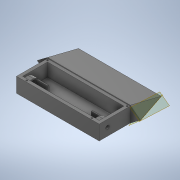
# Autodesk Inventor part: BodyWedgeV3
Saved by Autodesk Inventor 2020 (Build 240168000, 168)
## iProperties
Created: 2023-11-26
Part Number: BodyWedgeV3
Material: Thermoplastic Resin
Document SubType Name: Modeling
Designer: smz3rm
Density: 1.28 g/cm^3
Appearance: Smooth - Black
Mass: 333.31 g
Surface Area: 631.422 cm^2
Volume: 260.399 cm^3
Author: smz3rm
Autodesk Inventor part; units mm, degrees
ref_plane "YZ Plane" through (0, 0, 0) normal (1, 0, 0) x (0, 1, 0)
ref_plane "XZ Plane" through (0, 0, 0) normal (0, 1, 0) x (-1, 0, 0)
sketch "Sketch1" plane through (0, 0, 0) normal (0, 1, 0) x (-1, 0, 0)
  line L0 (80, 30) -> (-80, 30)
  line L1 (-80, 30) -> (-80, -30)
  line L2 (-80, -30) -> (80, -30)
  line L3 (80, -30) -> (80, 30)
  line L4 (80, 30) -> (-80, -30) construction
  line L5 (-80, 30) -> (80, -30) construction
  line L6 (0, -42) -> (0, 42) projected
  point P0 (0, 0)
  point P1 (-100, -30)
  point P2 (-80, -27)
  dimension "d0" = 160
  dimension "d1" = 60
  dimension "d32" = 20
  constraints: 12 end point, 2 midpoint, 2 parallel, 2 point on line, 1 horizontal, 1 perpendicular
  measures "d0" distance of L2.end L1.end
  measures "d1" distance of L1.end L0.end
  measures "d32" distance of L1.end point (-100, -30)
extrude "Extrusion1" add sketch "Sketch1" along normal blind 3
sketch "Sketch2" plane through (0, 3, 0) normal (0, 1, 0) x (1, 0, 0)
  line L0 (-80, 30) -> (-80, -30) projected
  line L1 (-80, -30) -> (80, -30) projected
  line L2 (80, -30) -> (80, 30) projected
  line L3 (74, -24) -> (-74, -24)
  line L4 (-74, -24) -> (-74, 24)
  line L5 (-74, 24) -> (74, 24)
  line L6 (74, 24) -> (74, -24)
  line L7 (74, -24) -> (-74, 24) construction
  line L8 (-74, -24) -> (74, 24) construction
  line L9 (80, 30) -> (-80, 30) projected
  point P0 (0, 0)
  dimension "d36" = 148
  dimension "d37" = 48
  constraints: 12 end point, 2 midpoint, 2 parallel, 1 horizontal, 1 perpendicular
  measures "d36" distance of L4.end L5.end
  measures "d37" distance between parallel lines of L5 L3
extrude "Extrusion2" add sketch "Sketch2" along normal blind 24
sketch "Sketch7" plane through (-74, 3, 24) normal (1, 0, 0) x (0, 0, -1)
  circle A0 centre (10, 12) radius 8
  line L0 (54, -3) -> (-6, -3) projected
  circle A1 centre (10, 12) radius 10
  line L1 (0, 12) -> (0, 0)
  line L2 (0, 12) -> (20, 12)
  line L3 (20, 12) -> (20, 0)
  line L4 (-6, -3) -> (-6, 24) projected
  line L5 (0, 0) -> (20, 0)
  line L6 (10, 22) -> (0, 22)
  line L7 (0, 0) -> (0, 24) projected
  line L8 (0, 12) -> (0, 22)
  point P0 (24, -3)
  point P1 (54, -3)
  dimension "MotorDiameter" = 16
  dimension "d18" = 15
  dimension "d20" = 2
  dimension "d40" = 20
  dimension "d62" = 10
  constraints: 12 end point, 3 horizontal, 3 point on circle, 2 centre point, 2 vertical, 1 perpendicular, 1 point on line
  measures "MotorDiameter" diameter of A0
  measures "d18" distance from line of L0 A0.centre
  measures "d20" radial gap between concentric circles of A0 A1
  measures "d40" distance between parallel lines of L3 L1
  measures "d62" distance of L6.start L6.end
extrude "Extrusion5" add sketch "Sketch7" along normal blind 11.25 contours L2 A1 A0 | A0 L2 A1 | L3 L5 L1 A1 | L7 L6 A1
sketch "Sketch8" plane through (-62.75, 3, 24) normal (1, 0, 0) x (0, 0, -1)
  arc A0 (20, 12) -> (10, 22) centre (10, 12) ccw projected
  circle A1 centre (10, 12) radius 8 projected
  line L0 (0, 0) -> (0, 22) projected
  line L1 (20, 0) -> (0, 0) projected
  line L2 (20, 0) -> (20, 12) projected
  circle A2 centre (10, 12) radius 7.75
  line L3 (10, 22) -> (0, 22) projected
  line L4 (0, 0) -> (0, 22) projected
  line L5 (4, 7.0946) -> (4, 17.2915)
  line L6 (10, 22) -> (0, 22) projected
  line L7 (16, 7.0946) -> (16, 17.2915)
  line L8 (16, 17.2915) -> (18.4853, 17.2915)
  arc A3 (20, 12) -> (10, 22) centre (10, 12) ccw projected
  line L9 (4, 17.2915) -> (0, 17.2915)
  point P0 (24, -3)
  point P1 (4, 27)
  point P2 (4, 16.9054)
  point P3 (16, 16.9054)
  dimension "d55" = 15.5
  dimension "d63" = 12
  dimension "d64" = 6
  constraints: 8 end point, 6 point on circle, 2 coincident, 2 perpendicular, 2 point on line, 1 centre point, 1 horizontal, 1 vertical
  measures "d55" diameter of A2
  measures "d63" distance between parallel lines of L7 L5
  measures "d64" distance from line of L5 point (10, 12)
extrude "Extrusion6" add sketch "Sketch8" along normal blind 20 contours L2 L1 L0 L9 A1 L8 A0 | A1 L5 A2 L7 | A2 L7 | L5 A2 picked at (9.114, 4.2488)
sketch "Sketch9" plane through (-74, 20, 20) normal (1, 0, 0) x (0, 0, -1)
  circle A0 centre (6, -5) radius 3.5
  line L0 (50, -20) -> (-10, -20) projected
  line L1 (-10, -20) -> (-10, 7) projected
  point P0 (20, -20)
  point P1 (44, -20)
  dimension "d27" = 7
  dimension "d28" = 15
  dimension "d41" = 16
  constraints: 1 centre point
  measures "d27" diameter of A0
  measures "d28" distance from line of L0 A0.centre
  measures "d41" distance from line of L1 A0.centre
extrude "Extrusion7" cut sketch "Sketch9" against normal up to surface (6 mm away)
mirror "Mirror2" about plane through (0, 0, 0) normal (1, 0, 0) of "Extrusion7", "Extrusion6", "Extrusion5"
sketch "Sketch15" plane through (80, 0, 30) normal (1, 0, 0) x (0, 0, -1)
  line L0 (60, 27) -> (0, 27) projected
  circle A0 centre (16, 15) radius 3.5 projected
  line L1 (0, 0) -> (60, 0) projected
  line L2 (60, 0) -> (60, 27) projected
  line L3 (0, 27) -> (60, 27) projected
  line L4 (0, 0) -> (0, 27) projected
  line L5 (60, 0) -> (60, 27) projected
  line L6 (120.0188, 15.0047) -> (60, 0)
  line L7 (60, 0) -> (60, 27) projected
  line L8 (60, 0) -> (60, 30)
  line L9 (60, 15) -> (120, 15)
  line L10 (60, 30) -> (120, 15)
  point P0 (30, 0)
  dimension "d104" = 30
  dimension "d105" = 15
  dimension "d106" = 60
  constraints: 8 end point, 1 horizontal, 1 midpoint, 1 point on line, 1 vertical
  measures "d104" distance of L1.end L8.end
  measures "d105" distance of L8.end L9.start
  measures "d106" distance of L9.start L9.end
extrude "Extrusion18" add sketch "Sketch15" against normal up to surface (160 mm away) contours L8 L10 L9 L2 | L9 L6 L2
ref_plane "Work Plane9" through (79, -4, -30) normal (0, 0, -1) x (-1, 0, 0)
sketch "Sketch23" plane through (79, -4, -30) normal (0, 0, -1) x (-1, 0, 0)
  line L0 (-1, 34) -> (-21, 19)
  line L1 (-21, 19) -> (-1, 19)
  line L2 (-21, 19) -> (-1, 4)
  line L3 (-1, 31) -> (159, 31) projected
  line L4 (-1, 34) -> (-1, 31) projected
  line L5 (-1, 34) -> (159, 34) projected
  line L6 (159, 34) -> (159, 31) projected
  line L7 (159, 4) -> (-1, 4) projected
  line L8 (-1, 4) -> (-1, 31) projected
  line L9 (159, 31) -> (-1, 31) projected
  line L10 (159, 4) -> (159, 31) projected
  point P0 (79, 4)
  dimension "d97" = 20
  dimension "d108" = 15
  constraints: 6 end point, 1 horizontal, 1 point on line
  measures "d97" distance of L0.end L1.end
  measures "d108" distance of L0.start L1.end
extrude "Extrusion19" add sketch "Sketch23" along normal blind 60 contours L4 L8 L1 L0 | L1 L8 L2
ref_plane "Work Plane4" through (100, 15, -30) normal (-0.5883, -0.7845, 0.1961) x (-0.8, 0.6, 0)
sketch "Sketch24" plane through (100, 15, -30) normal (-0.5883, -0.7845, 0.1961) x (-0.8, 0.6, 0)
  line L0 (-89.1969, -73.3175) -> (145.8797, -73.3175)
  line L1 (145.8797, -73.3175) -> (145.8797, 67.3582)
  line L2 (145.8797, 67.3582) -> (-89.1969, 67.3582)
  line L3 (-89.1969, 67.3582) -> (-89.1969, -73.3175)
  point P0 (71, -15.2971)
  constraints: 8 end point, 2 parallel, 1 horizontal, 1 perpendicular
extrude "Extrusion20" cut sketch "Sketch24" against normal blind 60
ref_plane "Work Plane5" through (80, 15, -90) normal (0.5883, -0.7845, -0.1961) x (0.3162, 0, 0.9487)
sketch "Sketch25" plane through (80, 15, -90) normal (0.5883, -0.7845, -0.1961) x (0.3162, 0, 0.9487)
  line L0 (-115.6054, 99.2741) -> (196.6383, 99.2741)
  line L1 (196.6383, 99.2741) -> (196.6383, -110.1424)
  line L2 (196.6383, -110.1424) -> (-115.6054, -110.1424)
  line L3 (-115.6054, -110.1424) -> (-115.6054, 99.2741)
  point P0 (60.0833, 91.1655)
  constraints: 8 end point, 2 parallel, 1 horizontal, 1 perpendicular
extrude "Extrusion21" cut sketch "Sketch25" along normal blind 60
mirror "Mirror10" about plane through (0, 0, 0) normal (1, 0, 0) of "Extrusion19", "Extrusion20", "Extrusion21"
sketch "Sketch26" plane through (0, 27, 0) normal (0, 1, 0) x (1, 0, 0)
  line L0 (-80, 30) -> (-80, -30) projected
  line L1 (-80, -30) -> (80, -30) projected
  line L2 (80, -30) -> (80, 30) projected
  line L3 (80, 30) -> (-80, 30) projected
  line L4 (-74, 24) -> (74, 24) projected
  line L5 (74, 24) -> (74, -24) projected
  line L6 (74, -24) -> (-74, -24) projected
  line L7 (-74, -24) -> (-74, 24) projected
  point P0 (0, 0)
extrude "Extrusion22" add sketch "Sketch26" along normal blind 1.4125
sketch "Sketch27" plane through (0, 28.4125, 0) normal (0, 1, 0) x (1, 0, 0)
  line L0 (-80, 30) -> (-80, -30) projected
  line L1 (-80, -30) -> (80, -30) projected
  line L2 (80, -30) -> (80, 30) projected
  line L3 (-80, 30) -> (80, 30) projected
  line L4 (-74, -24) -> (-74, 24) projected
  line L5 (-74, 24) -> (74, 24) projected
  line L6 (74, 24) -> (74, -24) projected
  line L7 (74, -24) -> (-74, -24) projected
  line L8 (80, -30) -> (80, 30) projected
  line L9 (80, -27) -> (-80, -27)
  line L10 (-80, 30) -> (-80, -30) projected
  line L11 (80, 27) -> (-80, 27)
  line L12 (-80, -30) -> (80, -30) projected
  line L13 (77, -30) -> (77, 30)
  circle A0 centre (63, -27) radius 1.45
  circle A1 centre (77, 27) radius 1.45
  line L14 (0, 114) -> (0, -54) projected
  circle A2 centre (-63, -27) radius 1.45
  circle A3 centre (-77, 27) radius 1.45
  point P0 (0, 0)
  dimension "d111" = 3
  dimension "d112" = 3
  dimension "d113" = 3
  dimension "d114" = 2.9
  dimension "d115" = 17
  dimension "d116" = 2.9
  constraints: 9 point on line, 6 end point, 4 centre point, 3 perpendicular, 2 symmetric about line, 2 other
  measures "d111" distance of L1.end L13.start
  measures "d112" distance of L1.end L9.start
  measures "d113" distance from line of L3 L11.start
  measures "d114" diameter of A0
  measures "d115" distance of L9.start A0.centre
  measures "d116" diameter of A1
extrude "Extrusion23" cut sketch "Sketch27" against normal blind 7 contours A3 L11 | L11 A3 | A2 L9 | L9 A2 | A1 L11 L13 | L13 L11 A1 | L11 L13 A1 | L11 A1 L13 | A0 L9 | L9 A0
ref_plane "Work Plane7" through (-100, 15, -30) normal (-0.5883, 0.7845, -0.1961) x (0.8, 0.6, 0)
ref_plane "Work Plane8" through (-80, 15, -90) normal (0.5883, 0.7845, 0.1961) x (-0.3162, 0, 0.9487)
equation "\"d0\" = Width"
equation "\"d1\" = Length"
equation "\"d32\" = -0.5 * Width + 0.5 * FullWidth"
equation "\"d2\" = BaseWallThickness"
equation "\"d36\" = Width - 2 * SideWallThickness"
equation "\"d37\" = Length - 2 * SideWallThickness"
equation "\"d5\" = Height - 2 * BaseWallThickness"
equation "\"d18\" = DriveMotorHeight"
equation "\"d20\" = DriveMotorMountThickness"
equation "\"d28\" = DriveMotorHeight"
equation "\"d41\" = SideWallThickness + DriveMotorMountThickness + 0.5 * MotorDiameter"
equation "\"d104\" = Height"
equation "\"d105\" = 0.5 * Height"
equation "\"d106\" = WedgeLength"
equation "\"d97\" = SideTriangleWidth"
equation "\"d98\" = WedgeLength"
equation "\"d100\" = WedgeLength"
equation "\"d102\" = WedgeLength"
equation "\"SideWallThickness\" = 6"
equation "\"BaseWallThickness\" = 3"
equation "\"Width\" = 160"
equation "\"Length\" = 60"
equation "\"Height\" = 30"
equation "\"DriveMotorHeight\" = 0.5 * Height"
equation "\"DriveMotorMountThickness\" = 2"
equation "\"WedgeLength\" = 60"
equation "\"SideTriangleWidth\" = 20"
equation "\"ScrewHoleDia\" = 2.9"
equation "\"ScrewDepth\" = 7"
equation "\"FullWidth\" = 200"
body "Solid1"
